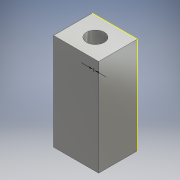
# Autodesk Inventor part: Solonoid Outside
Saved by Autodesk Inventor 2016 (Build 200138000, 138)
## iProperties
Created: 2016-05-08
Part Number: Solonoid Outside
Material: Generic
Document SubType Name: Modeling
Designer: Kenneth Daniel
Density: 1 g/cm^3
Appearance: Default
Author: Kenneth Daniel
Autodesk Inventor part; units mm, degrees
ref_plane "YZ Plane" through (0, 0, 0) normal (1, 0, 0) x (0, 1, 0)
ref_plane "XZ Plane" through (0, 0, 0) normal (0, 1, 0) x (-1, 0, 0)
ref_plane "XY Plane" through (0, 0, 0) normal (0, 0, 1) x (1, 0, 0)
sketch "Sketch1" plane through (0, 0, 0) normal (0, 1, 0) x (-1, 0, 0)
  line L0 (-7, 15) -> (-7, -15)
  line L1 (-7, -15) -> (7, -15)
  line L2 (7, -15) -> (7, 15)
  line L3 (7, 15) -> (-7, 15)
  line L4 (-7, 15) -> (7, -15) construction
  line L5 (-7, -15) -> (7, 15) construction
  point P0 (0, 0)
  dimension "d0" = 30
  dimension "d1" = 14
  constraints: 12 end point, 2 midpoint, 2 parallel, 1 perpendicular, 1 vertical
  measures "d0" distance of L0.start L0.end
  measures "d1" distance of L1.end L0.end
extrude "Extrusion1" add sketch "Sketch1" along normal blind 12
sketch "Sketch2" plane through (-7, 0, 15) normal (0, 0, 1) x (1, 0, 0)
  circle A0 centre (7, 6) radius 2.75
  point P0 (7, 0)
  dimension "d4" = 5.5
  constraints: 1 centre point
  measures "d4" diameter of A0
extrude "Extrusion2" cut sketch "Sketch2" against normal blind 25
sketch "Sketch3" plane through (0, 12, 0) normal (0, 1, 0) x (1, 0, 0)
  line L0 (7, -15) -> (7, 15) projected
  line L1 (7, 15) -> (-7, 15) projected
  line L2 (-7, 15) -> (-7, -15) projected
  line L3 (-7, -15) -> (7, -15) projected
  line L4 (-6, -14) -> (-6, 14)
  line L5 (-6, 14) -> (6, 14)
  line L6 (6, 14) -> (6, -14)
  line L7 (6, -14) -> (-6, -14)
  point P0 (0, 0)
  dimension "d7" = 1
  constraints: 8 end point, 3 other
  measures "d7" distance between parallel lines of L2 L4
sketch "Sketch4" plane through (0, 0, 0) normal (0, 0, 1) x (1, 0, 0)
  line L0 (7, 12) -> (-7, 12) projected
  line L1 (-7, 12) -> (7, 0)
  line L2 (7, 0) -> (7, 12) projected
  line L3 (7, 0) -> (7, 12)
  line L4 (7, 12) -> (-7, 0)
  line L5 (-7, 0) -> (-6, 0)
  line L6 (7, 0) -> (-7, 0) projected
  line L7 (-6, 0) -> (-6, 12)
  arc A0 (5.9979, 11.1411) -> (-6, 11.1429) centre (-0.0041, -9.3998) ccw
  line L8 (5.9979, 11.1411) -> (5.9979, 12)
  point P0 (0, 0)
  dimension "d8" = 1
  constraints: 12 end point, 6 point on line, 2 perpendicular, 2 point on circle, 1 centre point, 1 collinear
  measures "d8" distance of L4.end L5.end
extrude "Extrusion3" cut sketch "Sketch4" along normal mid plane 28 contours L8 A0 L0 | A0 L7 L0
body "Solid1"
